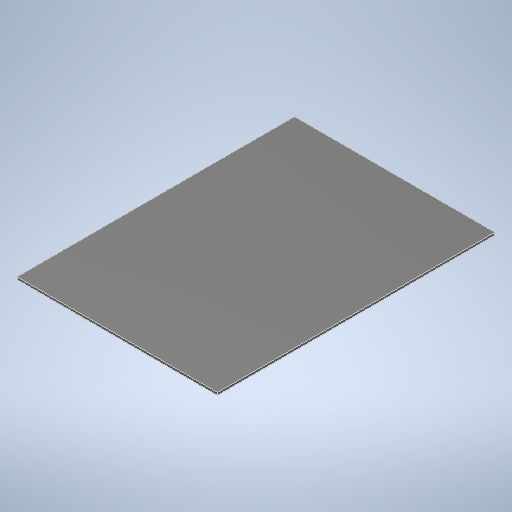
# Autodesk Inventor part: Bottom_Plate_Acryl
Saved by Autodesk Inventor 2026.2 (Build 302298010, 298A)
## iProperties
Created: 2026-03-27
Part Number: Bottom_Plate_Acryl
Material: Acetal Resin, Black
Document SubType Name: Modeling
Designer: chanh
Density: 1.425 g/cm^3
Appearance: Smooth - Black
Author: chanh
Autodesk Inventor part; units mm, degrees
ref_plane "YZ Plane" through (0, 0, 0) normal (1, 0, 0) x (0, 1, 0)
ref_plane "XZ Plane" through (0, 0, 0) normal (0, 1, 0) x (-1, 0, 0)
ref_plane "XY Plane" through (0, 0, 0) normal (0, 0, 1) x (1, 0, 0)
sketch "Sketch1" plane through (0, 0, 0) normal (0, 1, 0) x (-1, 0, 0)
  line L0 (195, 270) -> (-195, 270)
  line L1 (-195, 270) -> (-195, -270)
  line L2 (-195, -270) -> (195, -270)
  line L3 (195, -270) -> (195, 270)
  line L4 (195, 270) -> (-195, -270) construction
  line L5 (-195, 270) -> (195, -270) construction
  line L6 (-195, -10.9351) -> (-195, -110.9351)
  line L7 (195, -50) -> (195, 50)
  line L8 (-195, -200) -> (-195, -100)
  line L9 (195, -100) -> (195, -200)
  point P0 (0, 0)
  dimension "d0" = 390
  dimension "d1" = 540
  constraints: 20 end point, 4 parallel, 2 midpoint, 2 point on line, 1 horizontal, 1 perpendicular
  measures "d0" distance between parallel lines of L3 L1
  measures "d1" distance between parallel lines of L0 L2
extrude "Extrusion1" add sketch "Sketch1" along normal blind 5
body "Solid1"
